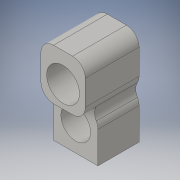
# Autodesk Inventor part: LED_mount
Saved by Autodesk Inventor 2016 (Build 200138000, 138)
## iProperties
Created: 2017-05-28
Part Number: LED_mount
Material: 一般
Document SubType Name: Modeling
Designer: kota
Density: 1 g/cm^3
Appearance: 既定
Author: kota
Autodesk Inventor part; units mm, degrees
ref_plane "YZ Plane" through (0, 0, 0) normal (1, 0, 0) x (0, 1, 0)
ref_plane "XZ Plane" through (0, 0, 0) normal (0, 1, 0) x (-1, 0, 0)
ref_plane "XY Plane" through (0, 0, 0) normal (0, 0, 1) x (1, 0, 0)
sketch "スケッチ1" plane through (0, 0, 0) normal (0, 1, 0) x (-1, 0, 0)
  line L0 (3.5, 4.25) -> (-3.5, 4.25)
  line L1 (-3.5, 4.25) -> (-3.5, -4.25)
  line L2 (-3.5, -4.25) -> (3.5, -4.25)
  line L3 (3.5, -4.25) -> (3.5, 4.25)
  line L4 (3.5, 4.25) -> (-3.5, -4.25) construction
  line L5 (-3.5, 4.25) -> (3.5, -4.25) construction
  point P0 (0, 0)
  dimension "d0" = 7
  dimension "d1" = 8.5
  constraints: 12 end point, 2 midpoint, 2 parallel, 1 horizontal, 1 perpendicular
  measures "d0" distance of L2.end L1.end
  measures "d1" distance of L0.end L1.end
extrude "押し出し1" add sketch "スケッチ1" along normal blind 15
sketch "スケッチ2" plane through (-3.5, 0, 4.25) normal (0, 0, 1) x (1, 0, 0)
  circle A0 centre (3.5, 4) radius 2.35
  line L0 (0, 0) -> (7, 0) projected
  line L1 (0, 0) -> (0, 15) projected
  circle A1 centre (3.5, 10.4) radius 2.6
  line L2 (0, 15) -> (7, 15) projected
  point P0 (3.5, 0)
  dimension "d4" = 4.7
  dimension "d5" = 4
  dimension "d6" = 3.5
  dimension "d7" = 5.2
  dimension "d8" = 4.6
  dimension "d9" = 3.5
  constraints: 2 centre point
  measures "d4" diameter of A0
  measures "d5" distance from line of L0 A0.centre
  measures "d6" distance from line of L1 A0.centre
  measures "d7" diameter of A1
  measures "d8" distance from line of L2 A1.centre
  measures "d9" distance from line of L1 A1.centre
extrude "押し出し2" cut sketch "スケッチ2" against normal blind 9
fillet "フィレット1" radius 2 1 edges at (3.5, 15, 0)
fillet "フィレット2" radius 2 1 edges at (-3.5, 15, 0)
sketch "スケッチ4" plane through (0, 0, 0) normal (0, -1, 0) x (1, 0, 0)
  line L0 (0, 6.3882) -> (0, -6.0661)
  line L1 (-5.5555, 5.25) -> (5.1337, 5.25)
  line L2 (-3.5, 4.25) -> (3.5, 4.25) projected
  point P0 (0, 0)
  dimension "d23" = 1
  constraints: 4 end point, 1 horizontal, 1 vertical, 2 other
  measures "d23" distance between parallel lines of L2 L1
sketch "スケッチ6" plane through (-3.5, 0, 4.25) normal (0, 0, 1) x (1, 0, 0)
  line L0 (0, 0) -> (7, 0) projected
  line L1 (0, 0) -> (7, 0)
  line L2 (7, 0) -> (7, 7)
  line L3 (7, 7) -> (0, 7)
  line L4 (0, 7) -> (0, 0)
  point P0 (3.5, 0)
  dimension "d27" = 7
  dimension "d28" = 7
  constraints: 8 end point, 2 parallel, 1 horizontal, 1 perpendicular
  measures "d27" distance of L3.end L2.end
  measures "d28" distance of L2.end L1.end
extrude "押し出し4" cut sketch "スケッチ6" against normal blind 2
sketch "スケッチ8" plane through (3.5, 0, -4.25) normal (0, 0, -1) x (-1, 0, 0)
  arc A0 (2, 7) -> (0, 5) centre (2, 5) ccw
  arc A1 (7, 5) -> (5, 7) centre (5, 5) ccw
  line L0 (0, 7) -> (7, 7) construction
  line L1 (0, 0) -> (7, 0) construction
  line L2 (0, 0) -> (0, 13) construction
  line L3 (7, 0) -> (7, 13) construction
  arc A2 (0, 9) -> (2, 7) centre (2, 9) ccw
  arc A3 (5, 7) -> (7, 9) centre (5, 9) ccw
  line L4 (0, 5) -> (0, 9)
  line L5 (7, 5) -> (7, 9)
  line L6 (7, 7) -> (7, 13) projected
  point P0 (3.5, 0)
  dimension "d33" = 2
  dimension "d34" = 7
  constraints: 8 point on circle, 7 tangent, 6 end point, 4 centre point, 4 symmetric about line, 2 collinear, 1 equal radius, 1 horizontal, 2 other
  measures "d33" radius of A0
  measures "d34" distance between parallel lines of L1 L0
extrude "押し出し5" cut sketch "スケッチ8" against normal blind 8.5
fillet "フィレット3" radius 2 2 edges at (1.5, 7, -1) (-1.5, 7, -1)
sketch "スケッチ9" plane through (-3.5, 0, 2.25) normal (0, 0, 1) x (1, 0, 0)
  arc A0 (7, 5) -> (6.7321, 6) centre (5, 5) ccw projected
  line L0 (7, 0) -> (7, 5) projected
  line L1 (7, 0) -> (0, 0) projected
  line L2 (0, 0) -> (0, 5) projected
  arc A1 (0.2679, 6) -> (0, 5) centre (2, 5) ccw projected
  arc A2 (0.2679, 6) -> (0.2679, 8) centre (-1.4641, 7) ccw projected
  arc A3 (0, 9) -> (0.2679, 8) centre (2, 9) ccw projected
  line L3 (0, 9) -> (0, 13) projected
  arc A4 (2, 15) -> (0, 13) centre (2, 13) ccw projected
  line L4 (5, 15) -> (2, 15) projected
  arc A5 (7, 13) -> (5, 15) centre (5, 13) ccw projected
  line L5 (7, 9) -> (7, 13) projected
  arc A6 (6.7321, 8) -> (7, 9) centre (5, 9) ccw projected
  arc A7 (6.7321, 8) -> (6.7321, 6) centre (8.4641, 7) ccw projected
  circle A8 centre (3.5, 10.4) radius 2.6 projected
  circle A9 centre (3.5, 4) radius 2.35 projected
  arc A10 (5, 7) -> (6.7321, 8) centre (5, 9) ccw projected
  line L6 (2, 7) -> (5, 7) projected
  arc A11 (0.2679, 8) -> (2, 7) centre (2, 9) ccw projected
  point P0 (3.5, 0)
